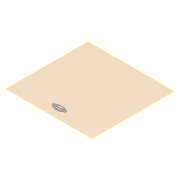
# Autodesk Inventor part: Part7
Saved by Autodesk Inventor 2014 (Build 180170000, 170)
## iProperties
Created: 2016-03-29
Part Number: Part7
Material: Stainless Steel
Document SubType Name: Modeling
Designer: admin
Density: 1 g/cm^3
Appearance: Semi-Polished
Author: admin
Autodesk Inventor part; units mm, degrees
ref_plane "YZ Plane" through (0, 0, 0) normal (1, 0, 0) x (0, 1, 0)
ref_plane "XZ Plane" through (0, 0, 0) normal (0, 1, 0) x (-1, 0, 0)
ref_plane "XY Plane" through (0, 0, 0) normal (0, 0, 1) x (1, 0, 0)
ref_plane "Work Plane1" through (0, 0, 0) normal (0, 0, 1) x (1, 0, 0)
sketch "Sketch1" plane through (0, 0, 0) normal (0, 0, 1) x (1, 0, 0)
  arc A0 (-148.6847, 77.7603) -> (-148.1357, 75.7112) centre (-147.3857, 77.0103) ccw projected
  line L0 (-148.6847, 77.7603) -> (-148.1847, 78.6263) projected
  line L1 (-148.1847, 78.6263) -> (-150.7828, 80.1263) projected
  line L2 (-150.7828, 80.1263) -> (-152.7828, 76.6622) projected
  arc A1 (-155.3809, 78.1622) -> (-152.7828, 76.6622) centre (-154.0818, 77.4122) ccw projected
  line L3 (-155.3809, 78.1622) -> (-158.3253, 79.8622) projected
  arc A2 (-156.8253, 82.4603) -> (-158.3253, 79.8622) centre (-157.5753, 81.1612) ccw projected
  line L4 (-156.8253, 82.4603) -> (-156.3253, 83.3263) projected
  line L5 (-156.3253, 83.3263) -> (-161.1751, 86.1263) projected
  arc A3 (-159.9251, 88.2913) -> (-161.1751, 86.1263) centre (-160.5501, 87.2088) ccw projected
  line L6 (-159.9251, 88.2913) -> (-155.0753, 85.4913) projected
  line L7 (-155.0753, 85.4913) -> (-151.5753, 91.5535) projected
  line L8 (-151.5753, 91.5535) -> (-156.4251, 94.3535) projected
  arc A4 (-155.1751, 96.5186) -> (-156.4251, 94.3535) centre (-155.8001, 95.4361) ccw projected
  line L9 (-155.1751, 96.5186) -> (-150.3253, 93.7186) projected
  line L10 (-150.3253, 93.7186) -> (-149.8253, 94.5846) projected
  arc A5 (-148.3253, 97.1827) -> (-149.8253, 94.5846) centre (-149.0753, 95.8836) ccw projected
  line L11 (-148.3253, 97.1827) -> (-145.3809, 95.4827) projected
  arc A6 (-142.7828, 93.9827) -> (-145.3809, 95.4827) centre (-144.0818, 94.7327) ccw projected
  line L12 (-142.7828, 93.9827) -> (-144.7828, 90.5186) projected
  line L13 (-144.7828, 90.5186) -> (-142.1847, 89.0186) projected
  line L14 (-142.1847, 89.0186) -> (-141.6847, 89.8846) projected
  arc A7 (-139.6357, 90.4336) -> (-141.6847, 89.8846) centre (-140.3857, 89.1346) ccw projected
  line L15 (-139.6357, 90.4336) -> (-134.9591, 87.7336) projected
  arc A8 (-134.4101, 85.6846) -> (-134.9591, 87.7336) centre (-135.7091, 86.4346) ccw projected
  line L16 (-134.4101, 85.6846) -> (-136.9101, 81.3545) projected
  line L17 (-136.9101, 81.3545) -> (-133.7924, 79.5545) projected
  arc A9 (-135.7924, 76.0904) -> (-133.7924, 79.5545) centre (-134.7924, 77.8224) ccw projected
  line L18 (-135.7924, 76.0904) -> (-138.9101, 77.8904) projected
  line L19 (-138.9101, 77.8904) -> (-141.4101, 73.5603) projected
  arc A10 (-143.4591, 73.0112) -> (-141.4101, 73.5603) centre (-142.7091, 74.3103) ccw projected
  line L20 (-143.4591, 73.0112) -> (-148.1357, 75.7112) projected
  arc A11 (141.6847, 89.8846) -> (139.6357, 90.4336) centre (140.3857, 89.1346) ccw projected
  line L21 (141.6847, 89.8846) -> (142.1847, 89.0186) projected
  line L22 (142.1847, 89.0186) -> (144.7828, 90.5186) projected
  line L23 (144.7828, 90.5186) -> (142.7828, 93.9827) projected
  arc A12 (145.3809, 95.4827) -> (142.7828, 93.9827) centre (144.0818, 94.7327) ccw projected
  line L24 (145.3809, 95.4827) -> (148.3253, 97.1827) projected
  arc A13 (149.8253, 94.5846) -> (148.3253, 97.1827) centre (149.0753, 95.8836) ccw projected
  line L25 (149.8253, 94.5846) -> (150.3253, 93.7186) projected
  line L26 (150.3253, 93.7186) -> (155.1751, 96.5186) projected
  arc A14 (156.4251, 94.3535) -> (155.1751, 96.5186) centre (155.8001, 95.4361) ccw projected
  line L27 (156.4251, 94.3535) -> (151.5753, 91.5535) projected
  line L28 (151.5753, 91.5535) -> (155.0753, 85.4913) projected
  line L29 (155.0753, 85.4913) -> (159.9251, 88.2913) projected
  arc A15 (161.1751, 86.1263) -> (159.9251, 88.2913) centre (160.5501, 87.2088) ccw projected
  line L30 (161.1751, 86.1263) -> (156.3253, 83.3263) projected
  line L31 (156.3253, 83.3263) -> (156.8253, 82.4603) projected
  arc A16 (158.3253, 79.8622) -> (156.8253, 82.4603) centre (157.5753, 81.1612) ccw projected
  line L32 (158.3253, 79.8622) -> (155.3809, 78.1622) projected
  arc A17 (152.7828, 76.6622) -> (155.3809, 78.1622) centre (154.0818, 77.4122) ccw projected
  line L33 (152.7828, 76.6622) -> (150.7828, 80.1263) projected
  line L34 (150.7828, 80.1263) -> (148.1847, 78.6263) projected
  line L35 (148.1847, 78.6263) -> (148.6847, 77.7603) projected
  arc A18 (148.1357, 75.7112) -> (148.6847, 77.7603) centre (147.3857, 77.0103) ccw projected
  line L36 (148.1357, 75.7112) -> (143.4591, 73.0112) projected
  arc A19 (141.4101, 73.5603) -> (143.4591, 73.0112) centre (142.7091, 74.3103) ccw projected
  line L37 (141.4101, 73.5603) -> (138.9101, 77.8904) projected
  line L38 (138.9101, 77.8904) -> (135.7924, 76.0904) projected
  arc A20 (133.7924, 79.5545) -> (135.7924, 76.0904) centre (134.7924, 77.8224) ccw projected
  line L39 (133.7924, 79.5545) -> (136.9101, 81.3545) projected
  line L40 (136.9101, 81.3545) -> (134.4101, 85.6846) projected
  arc A21 (134.9591, 87.7336) -> (134.4101, 85.6846) centre (135.7091, 86.4346) ccw projected
  line L41 (134.9591, 87.7336) -> (139.6357, 90.4336) projected
  line L42 (6, -167.6449) -> (6, -170.6449) projected
  line L43 (6, -170.6449) -> (10, -170.6449) projected
  arc A22 (10, -173.6449) -> (10, -170.6449) centre (10, -172.1449) ccw projected
  line L44 (10, -173.6449) -> (10, -177.0449) projected
  arc A23 (7, -177.0449) -> (10, -177.0449) centre (8.5, -177.0449) ccw projected
  line L45 (7, -177.0449) -> (6, -177.0449) projected
  line L46 (6, -177.0449) -> (6, -182.6449) projected
  arc A24 (3.5, -182.6449) -> (6, -182.6449) centre (4.75, -182.6449) ccw projected
  line L47 (3.5, -182.6449) -> (3.5, -177.0449) projected
  line L48 (3.5, -177.0449) -> (-3.5, -177.0449) projected
  line L49 (-3.5, -177.0449) -> (-3.5, -182.6449) projected
  arc A25 (-6, -182.6449) -> (-3.5, -182.6449) centre (-4.75, -182.6449) ccw projected
  line L50 (-6, -182.6449) -> (-6, -177.0449) projected
  line L51 (-6, -177.0449) -> (-7, -177.0449) projected
  arc A26 (-10, -177.0449) -> (-7, -177.0449) centre (-8.5, -177.0449) ccw projected
  line L52 (-10, -177.0449) -> (-10, -173.6449) projected
  arc A27 (-10, -170.6449) -> (-10, -173.6449) centre (-10, -172.1449) ccw projected
  line L53 (-10, -170.6449) -> (-6, -170.6449) projected
  line L54 (-6, -170.6449) -> (-6, -167.6449) projected
  line L55 (-6, -167.6449) -> (-7, -167.6449) projected
  arc A28 (-8.5, -166.1449) -> (-7, -167.6449) centre (-7, -166.1449) ccw projected
  line L56 (-8.5, -166.1449) -> (-8.5, -160.7449) projected
  arc A29 (-7, -159.2449) -> (-8.5, -160.7449) centre (-7, -160.7449) ccw projected
  line L57 (-7, -159.2449) -> (-2, -159.2449) projected
  line L58 (-2, -159.2449) -> (-2, -155.6449) projected
  arc A30 (2, -155.6449) -> (-2, -155.6449) centre (0, -155.6449) ccw projected
  line L59 (2, -155.6449) -> (2, -159.2449) projected
  line L60 (2, -159.2449) -> (7, -159.2449) projected
  arc A31 (8.5, -160.7449) -> (7, -159.2449) centre (7, -160.7449) ccw projected
  line L61 (8.5, -160.7449) -> (8.5, -166.1449) projected
  arc A32 (7, -167.6449) -> (8.5, -166.1449) centre (7, -166.1449) ccw projected
  line L62 (7, -167.6449) -> (6, -167.6449) projected
  arc A33 (174.3732, -22.7321) -> (67.5, 162.3777) centre (67.5, 38.9711) ccw projected
  line L63 (67.5, 162.3777) -> (-67.5, 162.3777) projected
  arc A34 (-67.5, 162.3777) -> (-174.3732, -22.7321) centre (-67.5, 38.9711) ccw projected
  line L64 (-174.3732, -22.7321) -> (-106.8732, -139.6455) projected
  arc A35 (-106.8732, -139.6455) -> (106.8732, -139.6455) centre (0, -77.9423) ccw projected
  line L65 (106.8732, -139.6455) -> (174.3732, -22.7321) projected
  circle A36 centre (160.7436, 60.4737) radius 2 projected
  circle A37 centre (132.7436, 108.9711) radius 2 projected
  circle A38 centre (-160.7436, 60.4737) radius 2 projected
  circle A39 centre (-132.7436, 108.9711) radius 2 projected
  circle A40 centre (28, -169.4449) radius 2 projected
  circle A41 centre (-28, -169.4449) radius 2 projected
  circle A42 centre (0, 0) radius 5 projected
  circle A43 centre (-28, -169.4449) radius 7
  circle A44 centre (28, -169.4449) radius 7
  line L66 (-12, -155.6449) -> (12, -155.6449)
  line L67 (12, -155.6449) -> (12, -185.6449)
  line L68 (12, -185.6449) -> (-12, -185.6449)
  line L69 (-12, -185.6449) -> (-12, -155.6449)
  line L70 (-30.5576, -162.9288) -> (-12, -155.6449)
  line L71 (-31.227, -175.6567) -> (-12, -185.6449)
  line L72 (31.227, -175.6567) -> (12, -185.6449)
  line L73 (30.5576, -162.9288) -> (12, -155.6449)
  line L74 (-7, -159.2449) -> (7, -159.2449)
  line L75 (8.5, -160.7449) -> (8.5, -166.1449)
  line L76 (7, -167.6449) -> (-7, -167.6449)
  line L77 (-8.5, -166.1449) -> (-8.5, -160.7449)
  line L78 (-10, -170.6449) -> (10, -170.6449)
  line L79 (10, -170.6449) -> (10, -177.0449)
  line L80 (10, -177.0449) -> (-10, -177.0449)
  line L81 (-10, -177.0449) -> (-10, -170.6449)
  arc A45 (-7, -159.2449) -> (-8.5, -160.7449) centre (-7, -160.7449) ccw
  arc A46 (-8.5, -166.1449) -> (-7, -167.6449) centre (-7, -166.1449) ccw
  arc A47 (7, -167.6449) -> (8.5, -166.1449) centre (7, -166.1449) ccw
  arc A48 (8.5, -160.7449) -> (7, -159.2449) centre (7, -160.7449) ccw
  circle A49 centre (-28, -169.4449) radius 2.15
  circle A50 centre (28, -169.4449) radius 2.15
  point P0 (0, 0)
  dimension "d2" = 14
  dimension "d3" = 14
  dimension "d5" = 30
  dimension "d6" = 2
  dimension "d7" = 2
  dimension "d8" = 1.5
  dimension "d16" = 4.3
  dimension "d17" = 4.3
  constraints: 32 end point, 12 point on circle, 12 tangent, 8 centre point, 6 parallel, 4 coincident, 3 equal radius, 3 horizontal, 3 perpendicular, 2 point on line, 1 midpoint
  measures "d2" diameter of A43
  measures "d3" diameter of A44
  measures "d5" distance of L66.end L67.end
  measures "d6" distance between parallel lines of L52 L69
  measures "d7" distance between parallel lines of L67 L44
  measures "d8" radius of A45
  measures "d16" diameter of A49
  measures "d17" diameter of A50
extrude "Extrusion1" add sketch "Sketch1" along normal blind 1.5 contours L62 A32 L61 A31 L60 L59 L66 L67 L68 L69 L58 L57 A29 L56 A28 L55 L54 L53 A27 L52 A26 L51 L50 A25 L49 L48 L47 A24 L46 L45 A23 L44 A22 L43 L42 | L42 L78 L54 L76 | A22 L79 | L81 A27 | A23 L80 | L80 A26 | L74 L58 L66 L59 | L46 A24 L47 L80 | L80 L49 A25 L50 | L73 A44 L72 L67 | L69 L71 A43 L70 | A44 | A43
fillet "Fillet1" radius 30 4 edges at (-12, -185.6449, 0.75) (12, -185.6449, 0.75) (-12, -155.6449, 0.75) (12, -155.6449, 0.75)
sketch "Sketch2" plane through (0, 0, 1.5) normal (0, 0, 1) x (1, 0, 0)
  line L0 (10, -177.0449) -> (-10, -177.0449) projected
  circle A0 centre (0, -182.0449) radius 1.5
  point P0 (0, 0)
  dimension "d12" = 3
  dimension "d13" = 5
  constraints: 1 centre point
  measures "d12" diameter of A0
  measures "d13" distance from line of L0 A0.centre
extrude "Extrusion2" cut sketch "Sketch2" against normal blind 10
body "Solid1"
